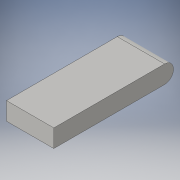
# Autodesk Inventor part: Battery
Saved by Autodesk Inventor 2016 (Build 200138000, 138)
## iProperties
Created: 2017-09-15
Part Number: Battery
Material: Generic
Document SubType Name: Modeling
Designer: Student
Density: 1 g/cm^3
Appearance: Default
Author: Student
Autodesk Inventor part; units mm, degrees
ref_plane "YZ Plane" through (0, 0, 0) normal (1, 0, 0) x (0, 1, 0)
ref_plane "XZ Plane" through (0, 0, 0) normal (0, 1, 0) x (-1, 0, 0)
ref_plane "XY Plane" through (0, 0, 0) normal (0, 0, 1) x (1, 0, 0)
sketch "Sketch1" plane through (0, 0, 0) normal (0, 1, 0) x (-1, 0, 0)
  line L0 (41.5198, 83.7231) -> (-25.7394, 83.7231)
  line L1 (-25.7394, 83.7231) -> (-25.7394, -86.4569)
  line L2 (-25.7394, -86.4569) -> (41.5198, -86.4569)
  line L3 (41.5198, -86.4569) -> (41.5198, 83.7231)
  point P0 (0, 0)
  dimension "d0" = 170.18
  dimension "d1" = 67.2592
  constraints: 8 end point, 2 parallel, 1 horizontal, 1 perpendicular
  measures "d0" distance of L2.end L0.start
  measures "d1" distance of L0.start L0.end
extrude "Extrusion1" add sketch "Sketch1" along normal blind 25.4
fillet "Fillet1" radius 12.7 2 edges at (-7.8902, 25.4, -86.4569) (-7.8902, 0, -86.4569)
body "Solid1"
